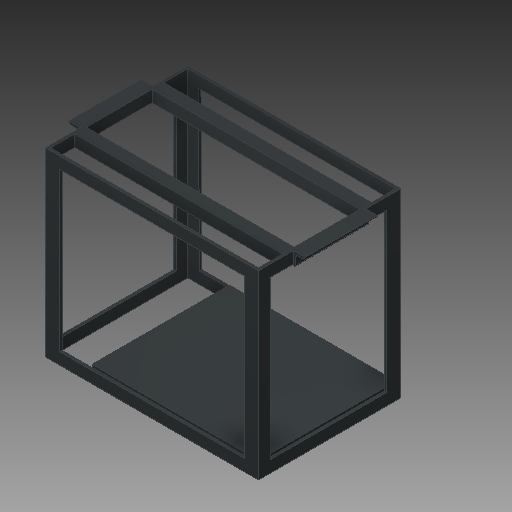
# Autodesk Inventor part: mesa
Saved by Autodesk Inventor 2019 (Build 230136000, 136)
## iProperties
Created: 2021-07-01
Part Number: mesa
Material: Hierro, fundido
Document SubType Name: Modeling
Designer: Usuario
Density: 7.15 g/cm^3
Appearance: Gris hierro
Author: Usuario
Autodesk Inventor part; units mm, degrees
ref_plane "YZ Plane" through (0, 0, 0) normal (1, 0, 0) x (0, 1, 0)
ref_plane "XZ Plane" through (0, 0, 0) normal (0, 1, 0) x (-1, 0, 0)
ref_plane "XY Plane" through (0, 0, 0) normal (0, 0, 1) x (1, 0, 0)
sketch "Boceto1" plane through (0, 0, 0) normal (0, 0, 1) x (1, 0, 0)
  line L0 (0, 0) -> (0, 544.715)
  line L1 (0, 544.715) -> (35, 544.715)
  line L2 (35, 509.715) -> (35, 0)
  line L3 (35, 0) -> (0, 0)
  line L4 (35, 544.715) -> (625, 544.715)
  line L5 (625, 544.715) -> (625, 509.715)
  line L6 (625, 509.715) -> (35, 509.715)
  line L7 (625, 509.715) -> (625, 0)
  line L8 (590, 0) -> (590, 509.715)
  line L9 (590, 0) -> (625, 0)
  line L10 (590, 0) -> (625, 0)
  line L11 (590, 509.715) -> (590, 0)
  line L12 (35, 0) -> (590, 0)
  line L13 (590, 0) -> (590, 35)
  line L14 (590, 35) -> (35, 35)
  line L15 (35, 544.715) -> (35, 509.715)
  line L16 (590, 509.715) -> (590, 544.715)
  dimension "d0" = 544.715
  dimension "d1" = 35
  dimension "d2" = 590
  dimension "d3" = 35
  dimension "d4" = 35
  dimension "d5" = 35
  constraints: 34 end point, 6 perpendicular, 4 point on line, 3 vertical, 2 collinear, 2 horizontal, 2 parallel
  measures "d0" distance of L0.start L0.end
  measures "d1" distance of L0.end L1.end
  measures "d2" distance of L1.end L4.end
  measures "d3" distance of L4.end L5.end
  measures "d4" distance of L7.end L8.start
  measures "d5" distance of L8.start L13.end
extrude "Extrusión1" add sketch "Boceto1" along normal blind 7.5 contours L0 L1 L15 L2 L3 | L2 L14 L8 L12 | L4 L16 L6 L15 | L8 L6 L7 L9 | L4 L5 L6 L16
ref_plane "Plano de trabajo1" through (0, 0, -617.5) normal (0, 0, -1) x (-1, 0, 0)
sketch "Boceto6" plane through (625, 0, 0) normal (1, 0, 0) x (0, 0, -1)
  line L0 (0, 0) -> (-7.5, 0) projected
  line L1 (-7.5, 0) -> (412.5, 0)
  line L2 (412.5, 0) -> (412.5, 544.715)
  line L3 (-7.5, 544.715) -> (-7.5, 0) projected
  line L4 (412.5, 544.715) -> (-7.5, 544.715)
  line L5 (-7.5, 544.715) -> (-7.5, 0)
  line L6 (-7.5, 544.715) -> (-7.5, 509.715)
  line L7 (-7.5, 509.715) -> (377.5, 509.715)
  line L8 (377.5, 509.715) -> (377.5, 35)
  line L9 (377.5, 35) -> (27.5, 35)
  line L10 (27.5, 35) -> (27.5, 509.715)
  dimension "d28" = 420
  dimension "d29" = 544.715
  dimension "d30" = 35
  dimension "d31" = 385
  dimension "d32" = 474.715
  dimension "d33" = 350
  constraints: 18 end point, 4 perpendicular, 2 collinear, 2 point on line, 1 vertical
  measures "d28" distance of L0.end L1.end
  measures "d29" distance of L1.end L2.end
  measures "d30" distance of L3.start L6.end
  measures "d31" distance of L6.end L7.end
  measures "d32" distance of L7.end L8.end
  measures "d33" distance of L8.end L9.end
extrude "Extrusión5" add sketch "Boceto6" along normal blind 7.5
sketch "Boceto7" plane through (625, 0, -412.5) normal (0, 0, -1) x (-1, 0, 0)
  line L0 (625, 544.715) -> (-7.5, 544.715) projected
  line L1 (-7.5, 544.715) -> (625, 544.715)
  line L2 (625, 544.715) -> (625, 0)
  line L3 (625, 0) -> (-7.5, 0) projected
  line L4 (625, 0) -> (-7.5, 0)
  line L5 (-7.5, 0) -> (-7.5, 544.715) projected
  line L6 (-7.5, 544.715) -> (-7.5, 0)
  line L7 (-7.5, 544.715) -> (-7.5, 509.715)
  line L8 (35, 509.715) -> (593, 509.715)
  line L9 (35, 35) -> (590, 35) projected
  line L10 (593, 509.715) -> (590, 35)
  line L11 (590, 35) -> (35, 35)
  line L12 (35, 35) -> (35, 509.715)
  dimension "d36" = 35
  dimension "d37" = 600.5
  constraints: 18 end point, 4 perpendicular, 1 collinear, 1 point on line, 1 vertical
  measures "d36" distance of L0.end L7.end
  measures "d37" distance of L7.end L8.end
extrude "Extrusión6" add sketch "Boceto7" along normal blind 7.5
sketch "Boceto8" plane through (0, 0, -412.5) normal (-1, 0, 0) x (0, 0, 1)
  line L0 (420, 544.715) -> (-7.5, 544.715) projected
  line L1 (-7.5, 544.715) -> (420, 544.715)
  line L2 (420, 544.715) -> (420, 0) projected
  line L3 (420, 544.715) -> (420, 0)
  line L4 (420, 0) -> (-7.5, 0)
  line L5 (412.5, 0) -> (0, 0) projected
  line L6 (-7.5, 0) -> (-7.5, 544.715)
  line L7 (-7.5, 35) -> (-7.5, 509.715) projected
  line L8 (-7.5, 544.715) -> (-7.5, 509.715)
  line L9 (385, 509.715) -> (385, 35) projected
  line L10 (35, 509.715) -> (385, 509.715)
  line L11 (385, 509.715) -> (385, 35)
  line L12 (35, 35) -> (35, 509.715) projected
  line L13 (385, 35) -> (35, 35)
  line L14 (35, 35) -> (35, 509.715)
  point P0 (144.8076, 0)
  point P1 (0, 415.0504)
  dimension "d40" = 35
  constraints: 18 end point, 5 perpendicular, 3 collinear, 1 point on line, 1 vertical, 2 other
  measures "d40" distance of L0.end L7.end
extrude "Extrusión7" add sketch "Boceto8" along normal blind 7.5
sketch "Boceto9" plane through (632.5, 544.715, 7.5) normal (0, 1, 0) x (1, 0, 0)
  line L0 (-640, 0) -> (0, 0) projected
  line L1 (-640, 0) -> (-640, 80)
  line L2 (-640, 0) -> (-640, 427.5) projected
  line L3 (-640, 80) -> (0, 80)
  line L4 (0, 80) -> (0, 115)
  line L5 (0, 115) -> (-640, 115)
  line L6 (-640, 115) -> (-640, 80)
  line L7 (0, 427.5) -> (-640, 427.5) projected
  line L8 (-640, 427.5) -> (-640, 347.5)
  line L9 (-640, 347.5) -> (0, 347.5)
  line L10 (0, 347.5) -> (0, 312.5)
  line L11 (0, 35) -> (0, 385) projected
  line L12 (0, 312.5) -> (-640, 312.5)
  line L13 (-640, 312.5) -> (-640, 347.5)
  point P0 (-632.5, 7.5)
  dimension "d43" = 80
  dimension "d44" = 640
  dimension "d45" = 35
  dimension "d46" = 640
  dimension "d47" = 80
  dimension "d48" = 640
  dimension "d49" = 35
  dimension "d50" = 640
  constraints: 20 end point, 6 point on line, 1 collinear, 1 horizontal, 1 perpendicular
  measures "d43" distance of L0.start L1.end
  measures "d44" distance of L1.end L3.end
  measures "d45" distance of L3.end L4.end
  measures "d46" distance of L4.end L5.end
  measures "d47" distance of L2.end L8.end
  measures "d48" distance of L8.end L9.end
  measures "d49" distance of L9.end L10.end
  measures "d50" distance of L10.end L12.end
extrude "Extrusión8" add sketch "Boceto9" against normal blind 35 contours L2 L5 L4 L3 | L2 L9 L10 L12
sketch "Boceto10" plane through (632.5, 0, 0) normal (1, 0, 0) x (0, 0, -1)
  line L0 (-7.5, 544.715) -> (-7.5, 0) projected
  line L1 (412.5, 544.715) -> (-7.5, 544.715) projected
  line L2 (-7.5, 544.715) -> (107.5, 544.715)
  line L3 (107.5, 544.715) -> (97.5, 544.715)
  line L4 (-7.5, 544.715) -> (420, 544.715) projected
  line L5 (97.5, 544.715) -> (97.5, 504.715)
  line L6 (420, 544.715) -> (420, 0) projected
  line L7 (420, 544.715) -> (315, 544.715)
  line L8 (315, 544.715) -> (315, 504.715)
  line L9 (315, 504.715) -> (97.5, 504.715)
  line L10 (97.5, 544.715) -> (315, 544.715)
  point P0 (0, 0)
  point P1 (305, 544.715)
  dimension "d53" = 115
  dimension "d54" = 10
  dimension "d55" = 40
  dimension "d56" = 105
  constraints: 14 end point, 2 perpendicular, 2 point on line, 1 collinear, 1 horizontal, 1 vertical
  measures "d53" distance of L0.start L2.end
  measures "d54" distance of L2.end L3.end
  measures "d55" distance of L3.end L5.end
  measures "d56" distance of L4.end L7.end
extrude "Extrusión9" add sketch "Boceto10" along normal blind 7.5
sketch "Boceto11" plane through (632.5, 504.715, -97.5) normal (0, 0, 1) x (1, 0, 0)
  line L0 (0, 40) -> (7.5, 40) projected
  line L1 (7.5, 40) -> (7.5, 32.5)
  line L2 (7.5, 40) -> (7.5, 0) projected
  line L3 (7.5, 0) -> (7.5, 40)
  line L4 (0, 40) -> (35, 40)
  line L5 (35, 40) -> (35, 32.5)
  line L6 (35, 32.5) -> (7.5, 32.5)
  line L7 (7.5, 32.5) -> (0, 32.5)
  line L8 (0, 5) -> (0, 40) projected
  line L9 (0, 32.5) -> (0, 40)
  point P0 (-632.5, -504.715)
  dimension "d59" = 7.5
  dimension "d64" = 35
  constraints: 14 end point, 2 collinear, 2 horizontal, 2 perpendicular, 1 point on line
  measures "d59" distance of L0.end L1.end
  measures "d64" distance of L0.start L4.end
extrude "Extrusión10" add sketch "Boceto11" against normal blind 217.5
fillet "Empalme1" radius 7.5 1 edges at (667.5, 537.215, -206.25)
fillet "Empalme2" radius 5 1 edges at (640, 537.215, -206.25)
fillet "Empalme3" radius 5 1 edges at (640, 504.715, -206.25)
sketch "Boceto14" plane through (-7.5, 0, -412.5) normal (-1, 0, 0) x (0, 0, 1)
  line L0 (-7.5, 544.715) -> (-7.5, 0) projected
  line L1 (97.5, 544.715) -> (-7.5, 544.715) projected
  line L2 (-7.5, 544.715) -> (97.5, 544.715)
  line L3 (97.5, 544.715) -> (97.5, 504.715)
  line L4 (97.5, 504.715) -> (315, 504.715)
  line L5 (315, 504.715) -> (315, 544.715)
  line L6 (315, 544.715) -> (97.5, 544.715)
  point P0 (412.5, 0)
  point P1 (0, 544.715)
  dimension "d76" = 105
  dimension "d77" = 40
  dimension "d78" = 217.5
  constraints: 10 end point, 4 perpendicular, 1 horizontal, 1 point on line
  measures "d76" distance of L0.start L1.start
  measures "d77" distance of L1.start L3.end
  measures "d78" distance of L3.end L4.end
extrude "Extrusión11" add sketch "Boceto14" along normal blind 7.5
sketch "Boceto15" plane through (-7.5, 504.715, -315) normal (0, 0, -1) x (-1, 0, 0)
  line L0 (0, 40) -> (0, 5) projected
  line L1 (0, 40) -> (35, 40)
  line L2 (35, 40) -> (35, 32.5)
  line L3 (35, 32.5) -> (0, 32.5)
  point P0 (-7.5, -504.715)
  dimension "d81" = 35
  dimension "d82" = 7.5
  constraints: 6 end point, 2 perpendicular, 1 horizontal, 1 point on line
  measures "d81" distance of L0.start L1.end
  measures "d82" distance of L1.end L2.end
extrude "Extrusión12" add sketch "Boceto15" against normal blind 217.5
fillet "Empalme4" radius 7.5 1 edges at (-42.5, 537.215, -206.25)
fillet "Empalme5" radius 5 1 edges at (-15, 537.215, -206.25)
fillet "Empalme6" radius 5 1 edges at (-15, 504.715, -206.25)
sketch "Boceto18" plane through (35, 35, -412.5) normal (0, 1, 0) x (1, 0, 0)
  line L0 (-35, 0) -> (590, 0) projected
  line L1 (590, 0) -> (550, 0)
  line L2 (550, 0) -> (490, 0)
  line L3 (490, 0) -> (90, 0)
  line L4 (90, 0) -> (90, -412.5)
  line L5 (590, -412.5) -> (-35, -412.5) projected
  line L6 (90, -412.5) -> (590, -412.5)
  line L7 (590, -412.5) -> (590, 0) projected
  line L8 (590, -412.5) -> (590, 0)
  line L9 (590, 0) -> (90, 0)
  point P0 (590, -144.8076)
  dimension "d90" = 40
  dimension "d91" = 60
  dimension "d92" = 400
  constraints: 14 end point, 4 point on line, 2 collinear, 2 perpendicular
  measures "d90" distance of L0.end L1.end
  measures "d91" distance of L1.end L2.end
  measures "d92" distance of L2.end L3.end
extrude "Extrusión13" add sketch "Boceto18" along normal mid plane 17.5
